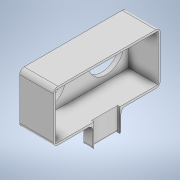
# Autodesk Inventor part: Ultaschal Sensor Gehäuse
Saved by Autodesk Inventor 2021 (Build 250183000, 183)
## iProperties
Created: 2021-06-22
Part Number: Ultaschal Sensor Gehäuse
Material: Generic
Document SubType Name: Modeling
Designer: Rami
Density: 1 g/cm^3
Appearance: Default
Author: Rami
Autodesk Inventor part; units mm, degrees
ref_plane "YZ Plane" through (0, 0, 0) normal (1, 0, 0) x (0, 1, 0)
ref_plane "XZ Plane" through (0, 0, 0) normal (0, 1, 0) x (-1, 0, 0)
ref_plane "XY Plane" through (0, 0, 0) normal (0, 0, 1) x (1, 0, 0)
sketch "Sketch1" plane through (0, 0, 0) normal (1, 0, 0) x (0, 1, 0)
  line L0 (0, 0) -> (20.7, 0)
  line L1 (20.7, 0) -> (20.7, -45.6)
  line L2 (20.7, -45.6) -> (0, -45.6)
  line L3 (0, -45.6) -> (0, 0)
  circle A0 centre (10.35, -9.5) radius 8
  circle A1 centre (10.35, -35.5) radius 8
  line L4 (21.7, -46.6) -> (21.7, 1)
  line L5 (21.7, 1) -> (-1, 1)
  line L6 (-1, 1) -> (-1, -46.6)
  line L7 (-1, -46.6) -> (21.7, -46.6)
  dimension "Breite" = 20.7
  dimension "Länge" = 45.6
  dimension "Kreise1" = 16
  dimension "BreiteBisKreise1" = 9.5
  dimension "LangeBisKreise" = 10.35
  dimension "KreiseCenter1BisKreiseCenter2" = 26
  dimension "Kreise2" = 16
  dimension "LangeBisKreise2" = 10.35
  dimension "d14" = 1
  constraints: 16 end point, 4 parallel, 2 centre point, 2 perpendicular, 1 horizontal, 3 other
  measures "Breite" distance of L1.end L2.end
  measures "Länge" distance of L0.end L1.end
  measures "Kreise1" diameter of A0
  measures "BreiteBisKreise1" distance from line of L0 A0.centre
  measures "LangeBisKreise" distance from line of L1 A0.centre
  measures "KreiseCenter1BisKreiseCenter2" distance of A1.centre A0.centre
  measures "Kreise2" diameter of A1
  measures "LangeBisKreise2" distance from line of L1 A1.centre
  measures "d14" distance between parallel lines of L1 L4
extrude "Extrusion1" add sketch "Sketch1" along normal blind 15 contours L0 L1 L2 L3 | A0 | A1
extrude "Extrusion2" add sketch "Sketch1" along normal up to surface (15 mm away) contours L7 L6 L5 L4
sketch "Sketch2" plane through (15, 0, 0) normal (1, 0, 0) x (0, 0, -1)
  line L0 (0, 20.7) -> (45.6, 20.7) projected
  line L1 (56.12, 0) -> (-10.52, 0) projected
  line L2 (45.6, 20.7) -> (45.6, 0) projected
  line L3 (0, -5.54) -> (0, 26.24) projected
  line L4 (0, 20.7) -> (45.6, 20.7)
  line L5 (45.6, 20.7) -> (45.6, 0)
  line L6 (45.6, 0) -> (0, 0)
  line L7 (0, 0) -> (0, 20.7)
  constraints: 8 end point, 2 parallel, 1 horizontal, 1 perpendicular
extrude "Extrusion3" cut sketch "Sketch2" against normal blind 13
extrude "Extrusion4" cut sketch "Sketch1" along normal blind 11 contours A0 | A1
sketch "Sketch3" plane through (15, 0, 0) normal (1, 0, 0) x (0, 0, -1)
  line L0 (45.6, 20.7) -> (45.6, 0) projected
  line L1 (45.6, 0) -> (0, 0) projected
  line L2 (0, 0) -> (0, 20.7) projected
  line L3 (0, 20.7) -> (45.6, 20.7) projected
  line L4 (-1, 21.7) -> (46.6, 21.7) projected
  line L5 (-1, -1) -> (-1, 21.7) projected
  line L6 (46.6, -1) -> (-1, -1) projected
  line L7 (46.6, 21.7) -> (46.6, -1) projected
  line L8 (0, 0) -> (0, 20.7) projected
  line L9 (0, 0) -> (16.5, 0)
  line L10 (45.6, 0) -> (0, 0) projected
  line L11 (45.6, 20.7) -> (45.6, 0) projected
  line L12 (45.6, 0) -> (29.1, 0)
  line L13 (-1, -1) -> (46.6, -1) projected
  line L14 (16.5, -1) -> (16.5, -10.5)
  line L15 (29.1, -1) -> (29.1, -10.5)
  line L16 (16.5, -10.5) -> (29.1, -10.5)
  dimension "d21" = 16.5
  dimension "d22" = 16.5
  dimension "d23" = 9.5
  dimension "d24" = 1
  dimension "d26" = 12.6
  constraints: 10 end point, 4 point on line, 3 perpendicular
  measures "d21" distance of L8.start L9.end
  measures "d22" distance of L0.end L12.end
  measures "d23" distance of L14.start L14.end
  measures "d24" distance of L9.end L14.start
  measures "d26" distance of L14.end L15.end
extrude "Extrusion5" add sketch "Sketch3" against normal blind 4 contours L6 L15 L16 L14
sketch "Sketch4" plane through (15, 0, 0) normal (1, 0, 0) x (0, 0, -1)
  line L0 (45.6, 20.7) -> (45.6, 0) projected
  line L1 (45.6, 0) -> (0, 0) projected
  line L2 (0, 0) -> (0, 20.7) projected
  line L3 (0, 20.7) -> (45.6, 20.7) projected
  line L4 (-1, 21.7) -> (46.6, 21.7) projected
  line L5 (-1, -1) -> (-1, 21.7) projected
  line L6 (16.5, -1) -> (-1, -1) projected
  line L7 (16.5, -1) -> (16.5, -10.5) projected
  line L8 (16.5, -10.5) -> (29.1, -10.5) projected
  line L9 (29.1, -10.5) -> (29.1, -1) projected
  line L10 (46.6, -1) -> (29.1, -1) projected
  line L11 (46.6, 21.7) -> (46.6, -1) projected
  line L12 (29.1, -10.5) -> (29.1, -1) projected
  line L13 (29.1, -10.5) -> (16.5, -10.5) projected
  line L14 (29.1, -1) -> (16.5, -1)
  line L15 (16.5, -1) -> (16.5, -10.5)
  line L16 (16.5, -10.5) -> (29.1, -10.5)
  line L17 (29.1, -10.5) -> (29.1, -1)
  line L18 (17, -1.5) -> (28.6, -1.5)
  line L19 (28.6, -1.5) -> (28.6, -10)
  line L20 (28.6, -10) -> (17, -10)
  line L21 (17, -10) -> (17, -1.5)
  line L22 (17, -1.5) -> (17, 0)
  line L23 (45.6, 0) -> (0, 0) projected
  line L24 (28.6, -1.5) -> (28.6, 0)
  line L25 (17, 0) -> (28.6, 0)
  line L26 (17, -10) -> (17, -10.5)
  line L27 (28.6, -10) -> (28.6, -10.5)
  dimension "d29" = 0.5
  constraints: 26 end point, 5 parallel, 4 perpendicular, 4 point on line, 1 collinear, 1 horizontal, 1 vertical, 3 other
  measures "d29" distance between parallel lines of L14 L18
extrude "Extrusion6" cut sketch "Sketch4" against normal blind 1 contours L24 L14 L22 L1 | L24 L18 L22 L14 | L19 L20 L21 L18 | L27 L8 L26 L20
fillet "Fillet1" radius 2 2 edges at (13, -1, -29.1) (13, -1, -16.5)
fillet "Fillet2" radius 2 4 edges at (7.5, -1, 1) (7.5, -1, -46.6) (7.5, 21.7, -46.6) (7.5, 21.7, 1)
fillet "Fillet3" radius 1 1 edges at (14, -10.5, -22.8)
fillet "Fillet4" radius 1 2 edges at (13, -10.5, -29.1) (13, -10.5, -16.5)
body "Solid1"
